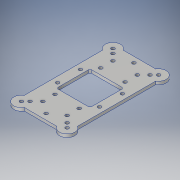
# Autodesk Inventor part: Piston Feed frame
Saved by Autodesk Inventor 2018.1 (Build 221171000, 171)
## iProperties
Created: 2013-10-18
Part Number: Piston Feed frame
Material: Aluminum 6061
Document SubType Name: Modeling
Designer: Gabriel Smolnycki
Density: 2.7 g/cm^3
Appearance: Aluminum - Flat
Mass: 78.6449 g
Surface Area: 182.425 cm^2
Volume: 29.1278 cm^3
Sending System: SolidWorks 2017
Last Author: Gabriel Smolnycki
Last Saved: 2017-09-14
Author: Gabriel Smolnycki
Autodesk Inventor part; units mm, degrees
ref_plane "YZ Plane" through (0, 0, 0) normal (1, 0, 0) x (0, 1, 0)
ref_plane "XZ Plane" through (0, 0, 0) normal (0, 1, 0) x (-1, 0, 0)
ref_plane "XY Plane" through (0, 0, 0) normal (0, 0, 1) x (1, 0, 0)
sketch "Sketch1" plane through (0, 0, 0) normal (0, 1, 0) x (-1, 0, 0)
  line L0 (-20, 22) -> (-22, 20)
  line L1 (-20, -22) -> (20, -22)
  line L2 (-35, 51.3397) -> (-35, -51.3397)
  arc A0 (35, 51.3397) -> (21.3397, 65) centre (30, 60) ccw
  arc A1 (21.3397, -65) -> (35, -51.3397) centre (30, -60) ccw
  line L3 (22, 20) -> (20, 22)
  line L4 (-22, 20) -> (-22, -20)
  line L5 (20, -22) -> (22, -20)
  arc A2 (-21.3397, 65) -> (-35, 51.3397) centre (-30, 60) ccw
  line L6 (35, -51.3397) -> (35, 51.3397)
  line L7 (20, 22) -> (-20, 22)
  line L8 (-22, -20) -> (-20, -22)
  arc A3 (-35, -51.3397) -> (-21.3397, -65) centre (-30, -60) ccw
  line L9 (21.3397, 65) -> (-21.3397, 65)
  line L10 (-21.3397, -65) -> (21.3397, -65)
  line L11 (22, -20) -> (22, 20)
  constraints: 24 end point, 8 equal length, 8 point on circle, 4 centre point, 4 horizontal, 4 vertical, 3 equal radius, 2 perpendicular
extrude "Extrusion1" add sketch "Sketch1" against normal blind 4.064
hole "Hole22" at (0, -4.064, 57.5) direction (0, 1, 0) diameter 4.5 depth 4.064
hole "Hole21" at (0, -4.064, -57.5) direction (0, 1, 0) diameter 4.5 depth 4.064
hole "Hole20" at (-16, 0, -46) direction (0, -1, 0) diameter 4.5 depth 4.064
hole "Hole19" at (-16, 0, -30) direction (0, -1, 0) diameter 4.5 depth 4.064
hole "Hole18" at (16, 0, -46) direction (0, -1, 0) diameter 4.5 depth 4.064
hole "Hole17" at (16, 0, -30) direction (0, -1, 0) diameter 4.5 depth 4.064
hole "Hole16" at (16, 0, 30) direction (0, -1, 0) diameter 4.5 depth 4.064
hole "Hole15" at (16, 0, 46) direction (0, -1, 0) diameter 4.5 depth 4.064
hole "Hole14" at (-16, 0, 30) direction (0, -1, 0) diameter 4.5 depth 4.064
hole "Hole13" at (-16, 0, 46) direction (0, -1, 0) diameter 4.5 depth 4.064
hole "Hole12" at (27.5, 0, -15) direction (0, -1, 0) diameter 4.5 depth 4.064
sketch "Sketch12" plane through (0, 0, 0) normal (0, 1, 0) x (-1, 0, 0)
  point P0 (-27.5, -15)
hole "Hole11" at (27.5, 0, 15) direction (0, -1, 0) diameter 4.5 depth 4.064
sketch "Sketch11" plane through (0, 0, 0) normal (0, 1, 0) x (-1, 0, 0)
  point P0 (16, 46)
hole "Hole10" at (-27.5, 0, -15) direction (0, -1, 0) diameter 4.5 depth 4.064
sketch "Sketch10" plane through (0, 0, 0) normal (0, 1, 0) x (-1, 0, 0)
  point P0 (16, 30)
hole "Hole9" at (-24.3431, 0, -54.3431) direction (0, -1, 0) diameter 4.5 depth 4.064
sketch "Sketch9" plane through (0, 0, 0) normal (0, 1, 0) x (-1, 0, 0)
  point P0 (-16, 46)
hole "Hole8" at (24.3431, 0, -54.3431) direction (0, -1, 0) diameter 4.5 depth 4.064
sketch "Sketch8" plane through (0, 0, 0) normal (0, 1, 0) x (-1, 0, 0)
  point P0 (-16, 30)
hole "Hole7" at (24.3431, 0, 54.3431) direction (0, -1, 0) diameter 4.5 depth 4.064
sketch "Sketch7" plane through (0, 0, 0) normal (0, 1, 0) x (-1, 0, 0)
  point P0 (-16, -30)
hole "Hole6" at (-24.3431, 0, 54.3431) direction (0, -1, 0) diameter 4.5 depth 4.064
sketch "Sketch6" plane through (0, 0, 0) normal (0, 1, 0) x (-1, 0, 0)
  point P0 (-16, -46)
hole "Hole5" at (-30, -4.064, 60) direction (0, 1, 0) diameter 4.5 depth 4.064
sketch "Sketch5" plane through (0, 0, 0) normal (0, 1, 0) x (-1, 0, 0)
  point P0 (16, -30)
hole "Hole4" at (30, -4.064, 60) direction (0, 1, 0) diameter 4.5 depth 4.064
sketch "Sketch4" plane through (0, 0, 0) normal (0, 1, 0) x (-1, 0, 0)
  point P0 (16, -46)
hole "Hole3" at (30, -4.064, -60) direction (0, 1, 0) diameter 4.5 depth 4.064
sketch "Sketch3" plane through (0, -4.064, 0) normal (0, -1, 0) x (1, 0, 0)
  point P0 (0, -57.5)
hole "Hole2" at (-30, -4.064, -60) direction (0, 1, 0) diameter 4.5 depth 4.064
sketch "Sketch2" plane through (0, -4.064, 0) normal (0, -1, 0) x (1, 0, 0)
  point P0 (0, 57.5)
hole "Hole1" at (-27.5, 0, 15) direction (0, -1, 0) diameter 4.5 depth 4.064
sketch "Sketch13" plane through (0, 0, 0) normal (0, 1, 0) x (-1, 0, 0)
  point P0 (-27.5, 15)
sketch "Sketch14" plane through (0, 0, 0) normal (0, 1, 0) x (-1, 0, 0)
  point P0 (27.5, -15)
sketch "Sketch15" plane through (0, 0, 0) normal (0, 1, 0) x (-1, 0, 0)
  point P0 (24.3431, -54.3431)
sketch "Sketch16" plane through (0, 0, 0) normal (0, 1, 0) x (-1, 0, 0)
  point P0 (-24.3431, -54.3431)
sketch "Sketch17" plane through (0, 0, 0) normal (0, 1, 0) x (-1, 0, 0)
  point P0 (-24.3431, 54.3431)
sketch "Sketch18" plane through (0, 0, 0) normal (0, 1, 0) x (-1, 0, 0)
  point P0 (24.3431, 54.3431)
sketch "Sketch19" plane through (0, -4.064, 0) normal (0, -1, 0) x (1, 0, 0)
  point P0 (-30, 60)
sketch "Sketch20" plane through (0, -4.064, 0) normal (0, -1, 0) x (1, 0, 0)
  point P0 (30, 60)
sketch "Sketch21" plane through (0, -4.064, 0) normal (0, -1, 0) x (1, 0, 0)
  point P0 (30, -60)
sketch "Sketch22" plane through (0, -4.064, 0) normal (0, -1, 0) x (1, 0, 0)
  point P0 (-30, -60)
sketch "Sketch23" plane through (0, 0, 0) normal (0, 1, 0) x (-1, 0, 0)
  point P0 (27.5, 15)
body "Solid3"
